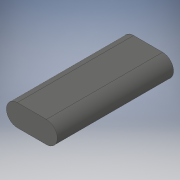
# Autodesk Inventor part: mockbattery
Saved by Autodesk Inventor 2018 (Build 220112000, 112)
## iProperties
Created: 2020-09-26
Part Number: mockbattery
Material: Generic
Document SubType Name: Modeling
Designer: Lveli
Density: 1 g/cm^3
Appearance: Gray
Author: Lveli
Autodesk Inventor part; units mm, degrees
ref_plane "YZ Plane" through (0, 0, 0) normal (1, 0, 0) x (0, 1, 0)
ref_plane "XZ Plane" through (0, 0, 0) normal (0, 1, 0) x (-1, 0, 0)
ref_plane "XY Plane" through (0, 0, 0) normal (0, 0, 1) x (1, 0, 0)
sketch "Sketch1" plane through (0, 0, 0) normal (0, 0, 1) x (1, 0, 0)
  line L0 (-12.7, 0) -> (12.7, 0) construction
  line L1 (-12.7, -9.525) -> (12.7, -9.525)
  line L2 (12.7, 9.525) -> (-12.7, 9.525)
  arc A0 (-12.7, 9.525) -> (-12.7, -9.525) centre (-12.7, 0) ccw
  arc A1 (12.7, -9.525) -> (12.7, 9.525) centre (12.7, 0) ccw
  point P0 (0, 0)
  dimension "d0" = 19.05
  dimension "d1" = 25.4
  constraints: 8 end point, 4 point on circle, 4 tangent, 2 centre point, 1 horizontal, 1 midpoint, 1 parallel
  measures "d0" diameter of A1
  measures "d1" distance of L0.start L0.end
extrude "Extrusion1" add sketch "Sketch1" along normal blind 101.6
body "Solid1"
